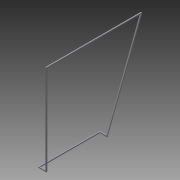
# Autodesk Inventor part: CatchFrameRight
Saved by Autodesk Inventor 2013 (Build 170138000, 138)
## iProperties
Created: 2014-01-24
Part Number: CatchFrameRight
Material: Generic
Document SubType Name: Modeling
Designer: Jarod
Density: 1 g/cm^3
d0: 0.250 in
d1: 15.000 in
d2: 0.250 in
d3: 0.00 deg
d4: 0.250 in
d5: 0.250 in
d6: 1.500 in
d7: 0.00 deg
d8: 0.250 in
d9: 22.000 in
d10: 0.250 in
d11: 0.00 deg
d16: 0.250 in
d17: 0.250 in
d18: 14.500 in
d19: 0.00 deg
d21: 8.500 in
d22: 0.00 deg
Author: Jarod
Autodesk Inventor part; units mm, degrees
ref_plane "YZ Plane" through (0, 0, 0) normal (1, 0, 0) x (0, 1, 0)
ref_plane "XZ Plane" through (0, 0, 0) normal (0, 1, 0) x (-1, 0, 0)
ref_plane "XY Plane" through (0, 0, 0) normal (0, 0, 1) x (1, 0, 0)
sketch "Sketch1" plane through (0, 0, 0) normal (1, 0, 0) x (0, 1, 0)
  line L0 (0, 0) -> (6.35, 0)
  line L1 (6.35, 0) -> (6.35, -381)
  line L2 (6.35, -381) -> (0, -381)
  line L3 (0, -381) -> (0, 0)
  dimension "d0" = 6.35
  dimension "d1" = 381
  constraints: 8 end point, 2 parallel, 1 horizontal, 1 perpendicular
  measures "d0" distance of L1.end L2.end
  measures "d1" distance of L0.end L1.end
extrude "Extrusion1" add sketch "Sketch1" along normal blind 6.35
sketch "Sketch2" plane through (6.35, 0, 0) normal (1, 0, 0) x (0, 0, -1)
  line L0 (0, 6.35) -> (0, 0) projected
  line L1 (0, 0) -> (381, 0) projected
  line L2 (381, 6.35) -> (0, 6.35) projected
  line L3 (0, 6.35) -> (6.35, 6.35)
  line L4 (6.35, 6.35) -> (6.35, 0)
  line L5 (6.35, 0) -> (0, 0)
  line L6 (0, 0) -> (0, 6.35)
  line L7 (381, 0) -> (374.65, 0)
  line L8 (374.65, 0) -> (374.65, 6.35)
  line L9 (374.65, 6.35) -> (381, 6.35)
  line L10 (381, 6.35) -> (381, 0)
  dimension "d4" = 6.35
  dimension "d5" = 6.35
  constraints: 16 end point, 4 parallel, 2 horizontal, 2 perpendicular, 2 point on line
  measures "d4" distance of L4.end L5.end
  measures "d5" distance of L8.end L9.end
extrude "Extrusion2" add sketch "Sketch2" along normal blind 38.1 contours L2 L4 L1 L0 | L2 L10 L1 L8
sketch "Sketch3" plane through (44.45, 0, 0) normal (1, 0, 0) x (0, 0, -1)
  line L0 (6.35, 0) -> (0, 0)
  line L1 (0, 0) -> (0, 558.8)
  line L2 (0, 558.8) -> (6.35, 558.8)
  line L3 (6.35, 558.8) -> (6.35, 0)
  dimension "d8" = 6.35
  dimension "d9" = 558.8
  constraints: 8 end point, 2 parallel, 1 horizontal, 1 perpendicular
  measures "d8" distance of L1.end L2.end
  measures "d9" distance of L0.end L1.end
extrude "Extrusion3" add sketch "Sketch3" along normal blind 6.35
sketch "Sketch5" plane through (44.45, 6.35, -6.35) normal (0, 0, -1) x (-1, 0, 0)
  line L0 (-6.35, 552.45) -> (0, 552.45)
  line L1 (0, 552.45) -> (0, 546.1)
  line L2 (0, 546.1) -> (-6.35, 546.1)
  line L3 (-6.35, 546.1) -> (-6.35, 552.45)
  point P0 (44.45, -6.35)
  dimension "d16" = 6.35
  dimension "d17" = 6.35
  constraints: 8 end point, 2 parallel, 1 horizontal, 1 perpendicular
  measures "d16" distance of L1.end L2.end
  measures "d17" distance of L0.end L1.end
extrude "Extrusion5" add sketch "Sketch5" along normal blind 368.3
sketch "Sketch7" plane through (44.45, 6.35, -374.65) normal (0, 0, -1) x (-1, 0, 0)
  line L0 (-6.35, 552.45) -> (-6.35, 546.1) projected
  line L1 (-6.35, 546.1) -> (0, 546.1) projected
  line L2 (0, 546.1) -> (0, 552.45) projected
  line L3 (0, 552.45) -> (-6.35, 552.45) projected
  point P0 (44.45, -6.35)
extrude "Extrusion6" add sketch "Sketch7" along normal blind 215.9
sketch "Sketch9" plane through (44.45, 0, 0) normal (1, 0, 0) x (0, 0, -1)
  line L0 (381, 0) -> (381, 6.35) projected
  line L1 (381, 6.35) -> (374.65, 6.35) projected
  line L2 (374.65, 6.35) -> (374.65, 0) projected
  line L3 (374.65, 0) -> (381, 0) projected
  line L4 (374.65, 6.35) -> (374.65, 558.8)
  line L5 (374.65, 6.35) -> (927.1, 6.35) construction
  line L6 (374.65, 558.8) -> (590.55, 558.8)
  line L7 (590.55, 558.8) -> (590.55, 552.45)
  line L8 (590.55, 552.45) -> (381, 6.35)
  line L9 (590.55, 558.8) -> (584.2, 558.8)
  line L10 (584.2, 558.8) -> (584.2, 552.45)
  line L11 (584.2, 552.45) -> (590.55, 552.45)
  line L12 (590.55, 552.45) -> (590.55, 558.8)
  line L13 (584.2, 552.45) -> (374.65, 6.35)
  point P0 (0, 0)
  dimension "d35" = 552.45
  dimension "d36" = 90
  dimension "d37" = 215.9
  dimension "d38" = 90
  dimension "d39" = 6.35
  dimension "d40" = 90
  dimension "d41" = 6.35
  dimension "d42" = 6.35
  constraints: 20 end point, 4 perpendicular, 3 parallel, 2 horizontal
  measures "d35" distance of L1.end L4.end
  measures "d36" angle of L5 L4
  measures "d37" distance of L4.end L6.end
  measures "d38" angle of L4 L6
  measures "d39" distance of L6.end L7.end
  measures "d40" angle of L6 L7
  measures "d41" distance of L11.end L10.end
  measures "d42" distance of L10.end L9.end
extrude "Extrusion8" add sketch "Sketch9" along normal blind 6.35 contours L3 L2 L1 L0 | L1 L13 L11 L8
body "Solid1"
